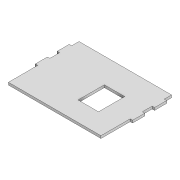
# Autodesk Inventor part: Top 2
Saved by Autodesk Inventor 2022 (Build 260153000, 153)
## iProperties
Created: 2022-06-16
Part Number: Top 2
Material: Generic
Document SubType Name: Modeling
Designer: ADMIN
Density: 1 g/cm^3
Appearance: Default
Author: ADMIN
Autodesk Inventor part; units mm, degrees
ref_plane "YZ Plane" through (0, 0, 0) normal (1, 0, 0) x (0, 1, 0)
ref_plane "XZ Plane" through (0, 0, 0) normal (0, 1, 0) x (-1, 0, 0)
ref_plane "XY Plane" through (0, 0, 0) normal (0, 0, 1) x (1, 0, 0)
sketch "Sketch1" plane through (0, 0, 0) normal (0, 1, 0) x (-1, 0, 0)
  line L0 (22.4826, 148.6372) -> (-167.5174, 148.6372)
  line L1 (-167.5174, 148.6372) -> (-167.5174, 3.6372)
  line L2 (-167.5174, 3.6372) -> (22.4826, 3.6372)
  line L3 (22.4826, 3.6372) -> (22.4826, 148.6372)
  line L4 (-167.5174, 88.6372) -> (-172.5174, 88.6372)
  line L5 (-172.5174, 88.6372) -> (-172.5174, 63.6372)
  line L6 (-172.5174, 63.6372) -> (-167.5174, 63.6372)
  line L7 (-167.5174, 63.6372) -> (-167.5174, 88.6372)
  line L8 (-167.5174, 43.6372) -> (-172.5174, 43.6372)
  line L9 (-172.5174, 43.6372) -> (-172.5174, 18.6372)
  line L10 (-172.5174, 18.6372) -> (-167.5174, 18.6372)
  line L11 (-167.5174, 18.6372) -> (-167.5174, 43.6372)
  line L12 (-72.5174, 148.6372) -> (-72.5174, 3.6372) construction
  line L13 (22.4826, 88.6372) -> (27.4826, 88.6372)
  line L14 (27.4826, 88.6372) -> (27.4826, 63.6372)
  line L15 (27.4826, 63.6372) -> (22.4826, 63.6372)
  line L16 (22.4826, 43.6372) -> (27.4826, 43.6372)
  line L17 (27.4826, 43.6372) -> (27.4826, 18.6372)
  line L18 (27.4826, 18.6372) -> (22.4826, 18.6372)
  point P0 (0, 0)
  dimension "d0" = 190
  dimension "d1" = 145
  dimension "d2" = 5
  dimension "d3" = 25
  dimension "d4" = 5
  dimension "d5" = 25
  dimension "d6" = 20
  dimension "d7" = 15
  constraints: 38 end point, 8 symmetric about line, 6 parallel, 3 horizontal, 3 perpendicular, 2 midpoint, 2 point on line
  measures "d0" distance of L2.end L1.end
  measures "d1" distance of L0.end L1.end
  measures "d2" distance of L6.end L5.end
  measures "d3" distance of L5.end L4.end
  measures "d4" distance of L10.end L9.end
  measures "d5" distance of L9.end L8.end
  measures "d6" distance between parallel lines of L8 L6
  measures "d7" distance from line of L1.end L10
extrude "Extrusion1" add sketch "Sketch1" along normal blind 5
sketch "Sketch2" plane through (0, 5, 0) normal (0, 1, 0) x (1, 0, 0)
  line L0 (-27.4826, -43.6372) -> (-22.4826, -43.6372) projected
  line L1 (-22.4826, -43.6372) -> (-22.4826, -63.6372) projected
  line L2 (-22.4826, -63.6372) -> (-27.4826, -63.6372) projected
  line L3 (-27.4826, -63.6372) -> (-27.4826, -88.6372) projected
  line L4 (-27.4826, -88.6372) -> (-22.4826, -88.6372) projected
  line L5 (-22.4826, -88.6372) -> (-22.4826, -148.6372) projected
  line L6 (-22.4826, -148.6372) -> (167.5174, -148.6372) projected
  line L7 (167.5174, -148.6372) -> (167.5174, -88.6372) projected
  line L8 (167.5174, -88.6372) -> (172.5174, -88.6372) projected
  line L9 (172.5174, -88.6372) -> (172.5174, -63.6372) projected
  line L10 (172.5174, -63.6372) -> (167.5174, -63.6372) projected
  line L11 (167.5174, -63.6372) -> (167.5174, -43.6372) projected
  line L12 (167.5174, -43.6372) -> (172.5174, -43.6372) projected
  line L13 (172.5174, -43.6372) -> (172.5174, -18.6372) projected
  line L14 (172.5174, -18.6372) -> (167.5174, -18.6372) projected
  line L15 (167.5174, -18.6372) -> (167.5174, -3.6372) projected
  line L16 (167.5174, -3.6372) -> (-22.4826, -3.6372) projected
  line L17 (-22.4826, -3.6372) -> (-22.4826, -18.6372) projected
  line L18 (-22.4826, -18.6372) -> (-27.4826, -18.6372) projected
  line L19 (-27.4826, -18.6372) -> (-27.4826, -43.6372) projected
  line L20 (80.5174, -108.6372) -> (122.5174, -108.6372)
  line L21 (122.5174, -108.6372) -> (122.5174, -54.6372)
  line L22 (122.5174, -54.6372) -> (80.5174, -54.6372)
  line L23 (80.5174, -54.6372) -> (80.5174, -108.6372)
  point P0 (0, 0)
  dimension "d10" = 42
  dimension "d11" = 54
  dimension "d12" = 45
  dimension "d13" = 40
  constraints: 8 end point, 2 parallel, 1 horizontal, 1 perpendicular
  measures "d10" distance of L22.end L21.end
  measures "d11" distance of L21.end L20.end
  measures "d12" distance between parallel lines of L7 L21
  measures "d13" distance between parallel lines of L6 L20
extrude "Extrusion2" cut sketch "Sketch2" against normal blind 5 contours L23 L22 L21 L20
body "Solid1"
